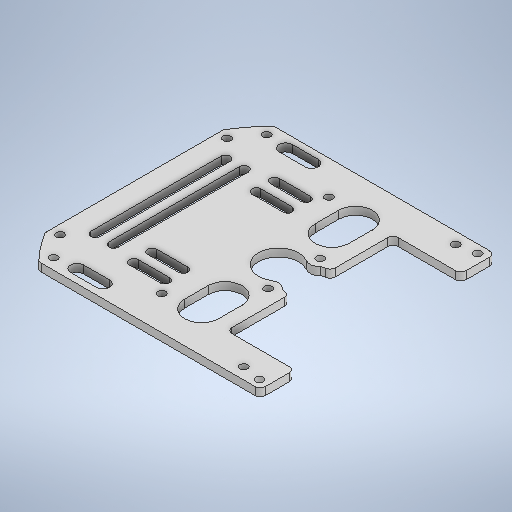
# Autodesk Inventor part: base_nivel2_V2
Saved by Autodesk Inventor 2025.3 (Build 293356030, 356C)
## iProperties
Created: 2025-04-02
Part Number: base_nivel2_V2
Material: Generic
Document SubType Name: Modeling
Designer: cdavi
Density: 1 g/cm^3
Appearance: Default
Mass: 22.5036 g
Surface Area: 171.079 cm^2
Volume: 22.5036 cm^3
Author: cdavi
Autodesk Inventor part; units mm, degrees
ref_plane "YZ Plane" through (0, 0, 0) normal (1, 0, 0) x (0, 1, 0)
ref_plane "XZ Plane" through (0, 0, 0) normal (0, 1, 0) x (-1, 0, 0)
ref_plane "XY Plane" through (0, 0, 0) normal (0, 0, 1) x (1, 0, 0)
sketch "Sketch1" plane through (0, 0, 0) normal (0, 1, 0) x (-1, 0, 0)
  circle A0 centre (0, 0) radius 54.1913 construction
  line L0 (0, 54.1913) -> (0, -54.1913) construction
  circle A1 centre (-34.5, 41.7906) radius 1.5
  line L1 (0, 0) -> (-54.1913, 0)
  circle A2 centre (-34.5, -41.7906) radius 1.5
  line L2 (-38, 52.7352) -> (-38, -52.7352)
  circle A3 centre (0, 0) radius 7.75
  circle A4 centre (0, 0) radius 65
  circle A5 centre (-34.5, -41.7906) radius 1.5
  line L3 (12.75, 32) -> (51.75, 32) construction
  line L4 (51.75, 32) -> (51.75, -32) construction
  line L5 (51.75, -32) -> (12.75, -32) construction
  line L6 (12.75, -32) -> (12.75, 32) construction
  circle A6 centre (0, 0) radius 70 construction
  line L7 (-45, 53.619) -> (-45, -53.619) construction
  line L8 (0, 0) -> (-34.5, 41.7906) construction
  circle A7 centre (-27.3, 40.619) radius 1.5
  circle A8 centre (-27.3, -40.619) radius 1.5
  circle A9 centre (51.75, -32) radius 1.5
  line L9 (51.75, -32) -> (55.2843, -34.1855)
  circle A10 centre (51.75, 32) radius 1.5
  circle A11 centre (12.75, 32) radius 1.5
  circle A12 centre (12.75, -32) radius 1.5
  circle A13 centre (45.3318, 40.817) radius 1.5
  circle A14 centre (45.3318, -40.817) radius 1.5
  line L10 (0, 29.5) -> (0, 20.5) construction
  line L11 (-6.5, 29.5) -> (-6.5, 20.5)
  line L12 (6.5, 20.5) -> (6.5, 29.5)
  arc A15 (6.5, 29.5) -> (-6.5, 29.5) centre (0, 29.5) ccw
  arc A16 (-6.5, 20.5) -> (6.5, 20.5) centre (0, 20.5) ccw
  line L13 (-6.5, -29.5) -> (-6.5, -20.5)
  line L14 (6.5, -20.5) -> (6.5, -29.5)
  arc A17 (-6.5, -29.5) -> (6.5, -29.5) centre (0, -29.5) ccw
  arc A18 (6.5, -20.5) -> (-6.5, -20.5) centre (0, -20.5) ccw
  line L15 (0, 0) -> (-12.842, 0) construction
  line L16 (-26.65, 0) -> (-17.65, 0)
  line L17 (0, 0) -> (45.3318, 40.817) construction
  line L18 (-7.75, 0) -> (-11.25, 0)
  line L19 (-11.25, 0) -> (-15.25, 0)
  line L20 (6.5, 21.5) -> (-6.5, 21.5)
  line L21 (37.25, 40) -> (27.25, 40) construction
  line L22 (37.25, 42.5) -> (27.25, 42.5)
  line L23 (27.25, 37.5) -> (37.25, 37.5)
  arc A19 (37.25, 37.5) -> (37.25, 42.5) centre (37.25, 40) ccw
  arc A20 (27.25, 42.5) -> (27.25, 37.5) centre (27.25, 40) ccw
  line L24 (46.9042, -45) -> (-38, -45)
  line L25 (46.9042, 45) -> (-38, 45)
  line L26 (-6.5, 21.5) -> (-6.6, 14.425) construction
  circle A21 centre (-6, 10) radius 1.5
  circle A22 centre (-6, -10) radius 1.5
  line L27 (37.25, -42.5) -> (27.25, -42.5)
  line L28 (27.25, -37.5) -> (37.25, -37.5)
  arc A23 (37.25, -42.5) -> (37.25, -37.5) centre (37.25, -40) ccw
  arc A24 (27.25, -37.5) -> (27.25, -42.5) centre (27.25, -40) ccw
  line L29 (-38, 31.869) -> (-12, 31.869)
  line L30 (-9.2486, 7.75) -> (-12, 7.75)
  line L31 (-12, 7.75) -> (-12, 31.869)
  arc A25 (-9.2486, 7.75) -> (-3.9457, 6.6704) centre (-6, 10.1432) ccw
  line L32 (-38, -31.869) -> (-12, -31.869)
  line L33 (-9.2486, -7.75) -> (-12, -7.75)
  line L34 (-12, -7.75) -> (-12, -31.869)
  arc A26 (-3.9457, -6.6704) -> (-9.2486, -7.75) centre (-6, -10.1432) ccw
  line L35 (32.25, -32) -> (32.25, 32)
  line L36 (45.25, 25) -> (45.25, -25) construction
  line L37 (47, 25) -> (47, -25)
  line L38 (43.5, -25) -> (43.5, 25)
  arc A27 (47, 25) -> (43.5, 25) centre (45.25, 25) ccw
  arc A28 (43.5, -25) -> (47, -25) centre (45.25, -25) ccw
  line L39 (38.25, 25) -> (38.25, -25) construction
  line L40 (36.5, 25) -> (36.5, -25)
  line L41 (40, -25) -> (40, 25)
  arc A29 (40, 25) -> (36.5, 25) centre (38.25, 25) ccw
  arc A30 (36.5, -25) -> (40, -25) centre (38.25, -25) ccw
  line L42 (28.5, -27) -> (16.5, -27) construction
  line L43 (28.5, -25.25) -> (16.5, -25.25)
  line L44 (16.5, -28.75) -> (28.5, -28.75)
  arc A31 (28.5, -28.75) -> (28.5, -25.25) centre (28.5, -27) ccw
  arc A32 (16.5, -25.25) -> (16.5, -28.75) centre (16.5, -27) ccw
  line L45 (32.25, 0) -> (12.75, 0)
  line L46 (22.5, 0) -> (22.5, -12.8588)
  line L47 (28.5, -20) -> (16.5, -20) construction
  line L48 (28.5, -18.25) -> (16.5, -18.25)
  line L49 (16.5, -21.75) -> (28.5, -21.75)
  arc A33 (28.5, -21.75) -> (28.5, -18.25) centre (28.5, -20) ccw
  arc A34 (16.5, -18.25) -> (16.5, -21.75) centre (16.5, -20) ccw
  line L50 (28.5, 25.25) -> (16.5, 25.25)
  line L51 (16.5, 28.75) -> (28.5, 28.75)
  arc A35 (28.5, 25.25) -> (28.5, 28.75) centre (28.5, 27) ccw
  arc A36 (16.5, 28.75) -> (16.5, 25.25) centre (16.5, 27) ccw
  line L52 (28.5, 18.25) -> (16.5, 18.25)
  line L53 (16.5, 21.75) -> (28.5, 21.75)
  arc A37 (28.5, 18.25) -> (28.5, 21.75) centre (28.5, 20) ccw
  arc A38 (16.5, 21.75) -> (16.5, 18.25) centre (16.5, 20) ccw
  line L54 (55.2843, -34.1855) -> (55.2843, 34.1855)
  circle A39 centre (0, 0) radius 48.9407 construction
  line L55 (0, 0) -> (-27.3, 40.619) construction
  point P0 (0, 7.75)
  point P1 (7.75, 0)
  point P2 (51.75, -16.0823)
  point P3 (51.75, -30.5)
  point P4 (50.25, -32)
  point P5 (43.7344, -32)
  point P6 (51.75, 16.0823)
  point P7 (43.7344, 32)
  point P8 (50.25, 32)
  point P9 (51.75, 30.5)
  point P10 (0, 25)
  point P11 (0, 14)
  point P12 (0, 36)
  point P13 (-45, -46.9042)
  point P14 (-45, 46.9042)
  point P15 (52.6522, 30.8017)
  point P16 (51.081, 33.3426)
  point P17 (51.081, -33.3426)
  point P18 (52.6522, -30.8017)
  point P19 (32.25, 40)
  point P20 (46.9042, 45)
  point P21 (45.25, 0)
  point P22 (51.75, 0)
  point P23 (38.25, 0)
  point P24 (22.5, -27)
  point P25 (22.5, -20)
  dimension "d101" = 97.8815
  dimension "d2" = 3
  dimension "d3" = 38
  dimension "d4" = 15.5
  dimension "d5" = 130
  dimension "d6" = 39
  dimension "d7" = 64
  dimension "d8" = 5
  dimension "d9" = 140
  dimension "d11" = 45
  dimension "d15" = 108.3827
  dimension "d16" = 39.541
  dimension "d17" = 3
  dimension "d18" = 17.7
  dimension "d19" = 13
  dimension "d20" = 3
  dimension "d21" = 4.1554
  dimension "d45" = 13
  dimension "d46" = 22
  dimension "d49" = 25
  dimension "d56" = 4.2947
  dimension "d58" = 48
  dimension "d59" = 61
  dimension "d60" = 3
  dimension "d68" = 1
  dimension "d70" = 5
  dimension "d71" = 5.5
  dimension "d72" = 10
  dimension "d75" = 45
  dimension "d76" = 7.0757
  dimension "d80" = 3
  dimension "d81" = 10
  dimension "d82" = 6
  dimension "d83" = 6
  dimension "d85" = 8.75
  dimension "d86" = 4.0349
  dimension "d87" = 3.2486
  dimension "d88" = 3.3296
  dimension "d89" = 50
  dimension "d90" = 3.5
  dimension "d91" = 6.5
  dimension "d92" = 3.5
  dimension "d93" = 50
  dimension "d94" = 7
  dimension "d95" = 3.5
  dimension "d96" = 12
  dimension "d97" = 27
  dimension "d98" = 3.5
  dimension "d99" = 7
  dimension "d100" = 12
  dimension "d102" = 33.905
  constraints: 124 end point, 61 point on circle, 39 centre point, 36 symmetric about line, 25 tangent, 15 point on line, 14 midpoint, 11 parallel, 10 coincident, 7 perpendicular, 6 vertical, 5 horizontal, 3 equal radius, 2 horizontal alignment, 1 line through centre, 1 vertical alignment, 17 other
  measures "d2" diameter of A1
  measures "d3" distance between parallel lines of L0 L2
  measures "d4" diameter of A3
  measures "d5" diameter of A4
  measures "d6" distance between parallel lines of L6 L4
  measures "d7" distance of L3.end L4.end
  measures "d8" distance from line of A3.end L6
  measures "d9" diameter of A6
  measures "d11" distance from line of L7 A3.centre
  measures "d15" diameter of A0
  measures "d16" angle of L0 L8
  measures "d17" diameter of A7
  measures "d18" horizontal distance of L7.start L55.end
  measures "d19" vertical distance of L7.start L55.end
  measures "d20" diameter of A9
  measures "d21" distance of L9.start L9.end
  measures "d45" distance between parallel lines of L11 L12
  measures "d46" distance of point (0, 14) point (0, 36)
  measures "d49" distance of point (0, 0) point (0, 25)
  measures "d58" angle of L0 L17
  measures "d59" distance of L15.start L17.end
  measures "d60" diameter of A13
  measures "d68" distance from line of L20 L10.end
  measures "d70" distance between parallel lines of L22 L23
  measures "d71" distance between parallel lines of L3 L23
  measures "d72" distance of L23.start L23.end
  measures "d75" distance from line of A4.centre L24
  measures "d76" distance of L20.end L26.end
  measures "d80" diameter of A21
  measures "d81" distance from line of L15 A21.centre
  measures "d82" distance from line of L0 A21.centre
  measures "d83" distance from line of A21.centre L31
  measures "d85" distance from line of L29 L55.end
  measures "d86" radius of A25
  measures "d87" horizontal distance of A21.centre L30.start
  measures "d88" vertical distance of A21.centre A25.end
  measures "d89" distance of L36.start L36.end
  measures "d90" distance between parallel lines of L38 L37
  measures "d91" distance of point (51.75, 0) point (45.25, 0)
  measures "d92" distance between parallel lines of L40 L41
  measures "d93" distance of L39.start L39.end
  measures "d94" distance of point (38.25, 0) point (45.25, 0)
  measures "d95" distance between parallel lines of L44 L43
  measures "d96" distance of L42.start L42.end
  measures "d97" distance between parallel lines of L45 L42
  measures "d98" distance between parallel lines of L48 L49
  measures "d99" distance of point (22.5, -27) point (22.5, -20)
  measures "d100" distance of L47.start L47.end
  measures "d102" angle of L0 L55
extrude "Extrusion1" add sketch "Sketch1" along normal blind 3 contours A25 L30 L31 L29 L2 L25 A4 L54 L24 L32 L34 L33 A26 A3
fillet "Fillet1" radius 2 14 edges at (38, 1.5, 45) (38, 1.5, -45) (-46.9042, 1.5, 45) (-46.9042, 1.5, -45) (12, 1.5, 7.75) (38, 1.5, 31.869) (12, 1.5, 31.869) (12, 1.5, -7.75) (9.2486, 1.5, -7.75) (9.2486, 1.5, 7.75) (-55.2843, 1.5, 34.1855) (-55.2843, 1.5, -34.1855) (12, 1.5, -31.869) (38, 1.5, -31.869)
body "Solid1"
